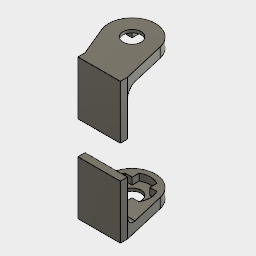
servo_bracket_ancle_1 (Autodesk Fusion 360 design; units mm, degrees)
Autodesk Fusion 360 part; units mm, degrees
sketch "スケッチ1" plane through (0, 0, 0) normal (0, 1, 0) x (1, 0, 0)
  line L0 (0, 0) -> (13, 0)
  line L1 (13, 0) -> (13, -2.2)
  line L2 (13, -2.2) -> (0, -2.2)
  line L3 (0, -2.2) -> (0, 0)
  line L4 (13, -2.2) -> (3, -2.2)
  line L5 (13, -2.2) -> (23, -2.2) construction
  line L6 (3, -2.2) -> (3, 11.4)
  line L7 (3, -2.2) -> (-10.6, -2.2) construction
  circle A0 centre (3, 11.4) radius 7.15
  line L8 (0, 0) -> (-3.6011, 8.6527)
  line L9 (13, 0) -> (9.9632, 13.0236)
  circle A1 centre (3, 11.4) radius 2.75
  dimension "d1" = 13
  dimension "d2" = 2.2
  dimension "d3" = 180
  dimension "d4" = 10
  dimension "d5" = 90
  dimension "d6" = 13.6
  dimension "d7" = 14.3
  dimension "d8" = 5.5
  constraint horizontal L0
  constraint vertical L1
  constraint horizontal L2
  constraint vertical L3
  constraint horizontal L5
  constraint horizontal L7
  constraint coincident A0
  constraint tangent A0 L8
  constraint tangent A0 L9
  constraint concentric A0 A1
  measures "d3" angle of L4 L5
  measures "d5" angle of L6 L7
  measures "d7" diameter of A0
  measures "d8" diameter of A1
sketch "スケッチ2" plane through (0, 0, 0) normal (0, 1, 0) x (1, 0, 0)
  line L0 (5.7, 8.7) -> (0.3, 8.7)
  line L1 (0.3, 8.7) -> (0.3, 14.1)
  line L2 (0.3, 14.1) -> (5.7, 14.1)
  line L3 (5.7, 14.1) -> (5.7, 8.7)
  line L4 (5.7, 8.7) -> (0.3, 14.1) construction
  line L5 (0.3, 8.7) -> (5.7, 14.1) construction
  circle A0 centre (3, 11.4) radius 5.55
  line L6 (5.7, 14.1) -> (5.7, 16.249)
  line L7 (5.7, 14.1) -> (7.849, 14.1)
  line L8 (0.3, 14.1) -> (0.3, 16.249)
  line L9 (0.3, 14.1) -> (-1.849, 14.1)
  line L10 (0.3, 8.7) -> (-1.849, 8.7)
  line L11 (0.3, 8.7) -> (0.3, 6.551)
  line L12 (5.7, 8.7) -> (5.7, 6.551)
  line L13 (5.7, 8.7) -> (7.849, 8.7)
  dimension "d9" = 5.4
  dimension "d10" = 5.4
  dimension "d11" = 11.1
  constraint perpendicular L0 L1
  constraint parallel L0 L2
  constraint parallel L1 L3
  constraint horizontal L0
  constraint coincident L4
  constraint coincident L5
  constraint coincident A0
  constraint perpendicular L2 L6
  constraint perpendicular L6 L7
  constraint perpendicular L7 L8
  constraint perpendicular L8 L9
  constraint perpendicular L1 L10
  constraint perpendicular L10 L11
  constraint perpendicular L0 L12
  constraint perpendicular L12 L13
  measures "d11" diameter of A0
extrude "押し出し1" add sketch "スケッチ1" against normal blind 16.425 contours L0 L2 L3 L6 | L0 L1 L2 L4 L6 makes body 1
extrude "押し出し2" add sketch "スケッチ1" against normal blind 3 contours L0 L6 A0 L8 | L0 L6 A0 L9 | A0 bodies 1
extrude "押し出し3" cut sketch "スケッチ2" against normal blind 5 contours L0 A0 L11 L12 | L0 L1 L2 L3 | L3 A0 L7 L13 | L1 A0 L9 L10 | L2 A0 L6 L8 bodies 1
extrude "押し出し4" add sketch "スケッチ2" against normal blind 0.9 contours L0 A0 L11 L12 | L0 L1 L2 L3 | L3 A0 L7 L13 | L1 A0 L9 L10 | L2 A0 L6 L8 bodies 1
extrude "押し出し5" cut sketch "スケッチ1" against normal blind 4 contours A1 bodies 1
fillet "フィレット1" radius 3 1 edges at (6.5, -3, 0) on bodies 1
ref_plane "作業平面1" through (6.5, -21.425, 1.1) normal (0, -1, 0) x (0, 0, -1)
mirror "ミラー1" about plane through (6.5, -21.425, 1.1) normal (0, -1, 0) of bodies 1 makes body 2
